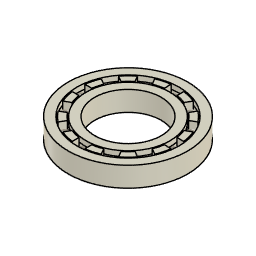
bearing_tutorial_60mm (Autodesk Fusion 360 design; units mm, degrees)
Autodesk Fusion 360 part; units mm, degrees
note: some values were not read from the file. Set by a fixed rule: which sketch regions a step uses.
sketch "Sketch1" plane through (0, 0, 0) normal (0, 0, 1) x (1, 0, 0)
  circle A0 centre (0, 0) radius 30
  circle A1 centre (0, 0) radius 25.6
  circle A2 centre (0, 0) radius 25.05
  circle A3 centre (0, 0) radius 21.65
  circle A4 centre (0, 0) radius 21.1
  circle A5 centre (0, 0) radius 16.7
  dimension "d1" = 60
  dimension "d2" = 4.4
  dimension "d3" = 0.55
  dimension "d4" = 3.4
  dimension "d5" = 0.55
  dimension "d6" = 4.4
  constraint coincident A0.centre A1.centre
  constraint concentric A0 A2
  constraint concentric A2 A3
  constraint concentric A2 A4
  constraint concentric A1 A5
  measures "d1" diameter of A0
  measures "d2" distance of A0 A1
  measures "d3" distance of A1 A2
  measures "d4" distance of A2 A3
  measures "d5" distance of A3 A4
  measures "d6" distance of A4 A5
extrude "Extrude1" add sketch "Sketch1" along normal blind 10 contours A0 makes body 1
extrude "Extrude2" add sketch "Sketch1" along normal blind 10 separate body contours A4 makes body 2
sketch "Sketch2" plane through (0, 0, 0) normal (0, 1, 0) x (1, 0, 0)
  line L0 (-30, -10) -> (30, -10) construction
  line L1 (25.6, -10) -> (-25.6, -10) construction
  line L2 (-21.1, -10) -> (21.1, -10) construction
  line L3 (16.7, -10) -> (-16.7, -10) construction
  line L4 (-30, 0) -> (30, 0) construction
  line L5 (21.1, -10) -> (21.1, 0) construction
  line L6 (25.6, -10) -> (25.6, 0) construction
  line L7 (25.6, -5) -> (21.1, -5) construction
  circle A0 centre (23.35, -5) radius 3.275
  dimension "d11" = 6.55
  constraint coincident L2.end L5.start
  constraint coincident L4 L5.end
  constraint perpendicular L4 L5
  constraint coincident L1.start L6.start
  constraint coincident L4 L6.end
  constraint perpendicular L4 L6
  constraint midpoint L6 L7.start
  constraint midpoint L5 L7.end
  constraint midpoint L7 A0.centre
  measures "d11" diameter of A0
revolve "Revolve1" cut sketch "Sketch2" angle 360 about axis through (0, 0, 1.75) along (0, 0, 1) bodies 1 2
extrude "Extrude3" add sketch "Sketch1" along normal blind 10 separate body contours A2 makes body 3
sketch "Sketch3" plane through (0, 0, 0) normal (0, 1, 0) x (1, 0, 0)
  line L0 (-25.05, -10) -> (25.05, -10) construction
  line L1 (0, 0) -> (0, -10) construction
  circle A0 centre (0, -5) radius 3.275
  line L2 (-3.175, -10) -> (-3.175, -5.8031)
  line L3 (3.175, -10) -> (3.175, -5.8031)
  line L4 (-3.175, -10) -> (3.175, -10)
  dimension "d15" = 6.55
  dimension "d16" = 3.175
  constraint coincident L1.start origin
  constraint midpoint L0 L1.end
  constraint midpoint L1 A0.centre
  constraint coincident L0 L2.start
  constraint coincident A0 L2.end
  constraint perpendicular L0 L2
  constraint symmetric L1 L2.start L3.start
  constraint symmetric L1 L2.end L3.end
  measures "d15" diameter of A0
  measures "d16" distance of L1 L2
extrude "Extrude4" cut sketch "Sketch3" along normal through all bodies 3
pattern_circular "C-Pattern1" count 12 over 360 about axis through (0, 0, 1.75) along (0, 0, 1) of "Extrude4"
sketch "Sketch4" plane through (0, 0, 0) normal (0, 1, 0) x (1, 0, 0)
  line L0 (-21.1, -10) -> (21.1, -10) construction
  line L1 (25.6, -10) -> (-25.6, -10) construction
  line L2 (-30, 0) -> (30, 0) construction
  line L3 (21.1, -10) -> (21.1, 0) construction
  line L4 (25.6, -10) -> (25.6, 0) construction
  line L5 (21.1, -5) -> (25.6, -5) construction
  circle A0 centre (23.35, -5) radius 3.175
  line L6 (23.35, -5) -> (23.35, -8.175)
  line L7 (23.35, -5) -> (23.35, -1.825)
  dimension "d20" = 6.35
  constraint coincident L0.end L3.start
  constraint coincident L2 L3.end
  constraint perpendicular L2 L3
  constraint coincident L1.start L4.start
  constraint coincident L2 L4.end
  constraint perpendicular L2 L4
  constraint midpoint L3 L5.start
  constraint midpoint L4 L5.end
  constraint midpoint L5 A0.centre
  constraint coincident A0.centre L6.start
  constraint coincident A0 L6.end
  constraint perpendicular L5 L6
  constraint coincident A0 L7.end
  constraint perpendicular L5 L7
  measures "d20" diameter of A0
revolve "Revolve2" add sketch "Sketch4" angle 360 about axis through (23.35, 0, 5) along (0, 0, 1) separate body contours A0 L6 L7 picked at (25.4559, -5.1506) makes body 4
pattern_circular "C-Pattern2" count 12 over 360 about axis through (0, 0, 1.75) along (0, 0, 1) of bodies 4 makes body 5 at (22.9478, 10.1011, 5.4144) makes body 6 at (14.8228, 20.2217, 4.5856) makes body 7 at (2.7261, 24.9239, 4.5856) makes body 8 at (-10.1011, 22.9478, 5.4144) makes body 9 at (-17.4956, 13.2489, 5.4144) makes body 10 at (-21.7761, 2.7261, 4.5856) makes body 11 at (-22.9478, -10.1011, 4.5856) makes body 12 at (-13.2489, -17.4956, 5.4144) makes body 13 at (-2.7261, -24.9239, 4.5856) makes body 14 at (10.1011, -22.9478, 5.4144) makes body 15 at (17.4956, -13.2489, 4.5856)
equation "d11 = ( 25.4 / 4 ) * 1 mm + 0.2 mm"
equation "d15 = ( 25.4 / 4 ) * 1 mm + 0.2 mm"
equation "d16 = ( 25.4 / 4 / 2 ) * 1 mm"
equation "d20 = ( 25.4 / 4 ) * 1 mm"
named bodies: "outer", "inner", "middle"
